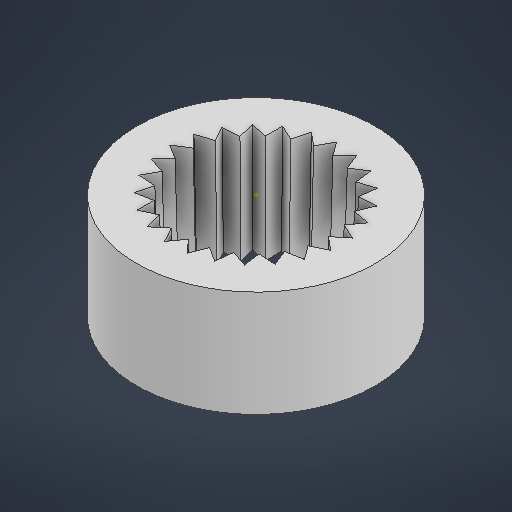
# Autodesk Inventor part: OMG_servo_head(1deg)
Saved by Autodesk Inventor 2026.1 (Build 301233020, 233B)
## iProperties
Created: 2026-02-22
Part Number: OMG_servo_head(1deg)
Material: Generic
Document SubType Name: Modeling
Designer: Lars
Density: 1 g/cm^3
Appearance: Default
Author: Lars
Autodesk Inventor part; units mm, degrees
ref_plane "YZ Plane" through (0, 0, 0) normal (1, 0, 0) x (0, 1, 0)
ref_plane "XZ Plane" through (0, 0, 0) normal (0, 1, 0) x (-1, 0, 0)
ref_plane "XY Plane" through (0, 0, 0) normal (0, 0, 1) x (1, 0, 0)
sketch "Sketch1" plane through (0, 0, 0) normal (0, 1, 0) x (-1, 0, 0)
  circle A0 centre (0, 0) radius 3.125 construction
  circle A1 centre (0, 0) radius 2.625 construction
  line L0 (3.125, 0) -> (2.6043, 0.329)
  line L1 (3.125, 0) -> (2.6043, -0.329)
  line L2 (3.125, 0) -> (2.625, 0) construction
  line L3 (3.0268, 0.7772) -> (2.4407, 0.9663)
  line L4 (3.0268, 0.7772) -> (2.6043, 0.329)
  line L5 (2.7385, 1.5055) -> (2.1237, 1.5429)
  line L6 (2.7385, 1.5055) -> (2.4407, 0.9663)
  line L7 (2.278, 2.1392) -> (1.6732, 2.0226)
  line L8 (2.278, 2.1392) -> (2.1237, 1.5429)
  line L9 (1.6745, 2.6385) -> (1.1177, 2.3752)
  line L10 (1.6745, 2.6385) -> (1.6732, 2.0226)
  line L11 (0.9657, 2.9721) -> (0.4919, 2.5785)
  line L12 (0.9657, 2.9721) -> (1.1177, 2.3752)
  line L13 (0.1962, 3.1188) -> (-0.1648, 2.6198)
  line L14 (0.1962, 3.1188) -> (0.4919, 2.5785)
  line L15 (-0.5856, 3.0696) -> (-0.8112, 2.4965)
  line L16 (-0.5856, 3.0696) -> (-0.1648, 2.6198)
  line L17 (-1.3306, 2.8276) -> (-1.4065, 2.2164)
  line L18 (-1.3306, 2.8276) -> (-0.8112, 2.4965)
  line L19 (-1.9919, 2.4079) -> (-1.9135, 1.7969)
  line L20 (-1.9919, 2.4079) -> (-1.4065, 2.2164)
  line L21 (-2.5282, 1.8368) -> (-2.3003, 1.2646)
  line L22 (-2.5282, 1.8368) -> (-1.9135, 1.7969)
  line L23 (-2.9056, 1.1504) -> (-2.5425, 0.6528)
  line L24 (-2.9056, 1.1504) -> (-2.3003, 1.2646)
  line L25 (-3.1004, 0.3917) -> (-2.625, 0)
  line L26 (-3.1004, 0.3917) -> (-2.5425, 0.6528)
  line L27 (-3.1004, -0.3917) -> (-2.5425, -0.6528)
  line L28 (-3.1004, -0.3917) -> (-2.625, 0)
  line L29 (-2.9056, -1.1504) -> (-2.3003, -1.2646)
  line L30 (-2.9056, -1.1504) -> (-2.5425, -0.6528)
  line L31 (-2.5282, -1.8368) -> (-1.9135, -1.7969)
  line L32 (-2.5282, -1.8368) -> (-2.3003, -1.2646)
  line L33 (-1.992, -2.4079) -> (-1.4065, -2.2164)
  line L34 (-1.992, -2.4079) -> (-1.9135, -1.7969)
  line L35 (-1.3306, -2.8276) -> (-0.8112, -2.4965)
  line L36 (-1.3306, -2.8276) -> (-1.4065, -2.2164)
  line L37 (-0.5856, -3.0696) -> (-0.1648, -2.6198)
  line L38 (-0.5856, -3.0696) -> (-0.8112, -2.4965)
  line L39 (0.1962, -3.1188) -> (0.4919, -2.5785)
  line L40 (0.1962, -3.1188) -> (-0.1648, -2.6198)
  line L41 (0.9657, -2.9721) -> (1.1177, -2.3752)
  line L42 (0.9657, -2.9721) -> (0.4919, -2.5785)
  line L43 (1.6745, -2.6385) -> (1.6732, -2.0226)
  line L44 (1.6745, -2.6385) -> (1.1177, -2.3752)
  line L45 (2.278, -2.1392) -> (2.1237, -1.5429)
  line L46 (2.278, -2.1392) -> (1.6732, -2.0226)
  line L47 (2.7385, -1.5055) -> (2.4407, -0.9663)
  line L48 (2.7385, -1.5055) -> (2.1237, -1.5429)
  line L49 (3.0268, -0.7772) -> (2.6043, -0.329)
  line L50 (3.0268, -0.7772) -> (2.4407, -0.9663)
  circle A2 centre (0, 0) radius 4.5
  point P0 (2.6043, -0.329)
  point P1 (2.4407, 0.9663)
  point P2 (-0.1648, 2.6198)
  point P3 (-2.625, 0)
  point P4 (-0.1648, -2.6198)
  point P5 (2.1237, -1.5429)
  dimension "d0" = 6.25
  dimension "d1" = 0.5
  dimension "d3" = 0.5
  dimension "d6" = 360
  dimension "d11" = 9
  constraints: 102 end point, 3 coincident, 3 point on circle, 2 centre point, 1 horizontal, 1 horizontal alignment, 129 other
  measures "d3" distance of L0.start L2.end
  measures "d11" diameter of A2
extrude "Extrusion1" add sketch "Sketch1" along normal blind 4 contours L1 L49 L50 L47 L48 L45 L46 L43 L44 L41 L42 L39 L40 L37 L38 L35 L36 L33 L34 L31 L32 L29 L30 L27 L28 L25 L26 L23 L24 L21 L22 L19 L20 L17 L18 L15 L16 L13 L14 L11 L12 L9 L10 L7 L8 L5 L6 L3 L4 L0 | A2
extrude "Extrusion2" cut sketch "Sketch1" along normal blind 4 draft 1 contours L1 L49 L50 L47 L48 L45 L46 L43 L44 L41 L42 L39 L40 L37 L38 L35 L36 L33 L34 L31 L32 L29 L30 L27 L28 L25 L26 L23 L24 L21 L22 L19 L20 L17 L18 L15 L16 L13 L14 L11 L12 L9 L10 L7 L8 L5 L6 L3 L4 L0
sketch "Sketch3" plane through (0, 4, 0) normal (0, 1, 0) x (1, 0, 0)
  point P0 (0, 0)
equation "\"d3\" = d1"
body "Solid1"
